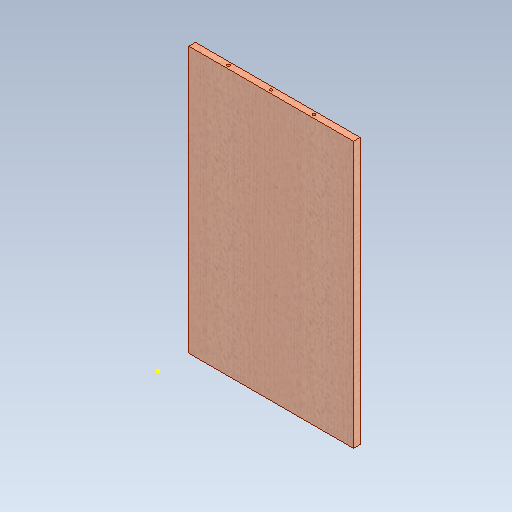
# Autodesk Inventor part: LateralInteriorCajoneras
Saved by Autodesk Inventor 2020.3 (Build 243373000, 373)
## iProperties
Created: 2020-10-30
Part Number: LateralInteriorCajoneras
Material: Madera (roble)
Document SubType Name: Modeling
Designer: codig
Density: 0.76 g/cm^3
Appearance: Roble blanco - Natural brillo medio
Author: codig
Autodesk Inventor part; units mm, degrees
ref_plane "YZ Plane" through (0, 0, 0) normal (1, 0, 0) x (0, 1, 0)
ref_plane "XZ Plane" through (0, 0, 0) normal (0, 1, 0) x (-1, 0, 0)
ref_plane "XY Plane" through (0, 0, 0) normal (0, 0, 1) x (1, 0, 0)
sketch "Boceto1" plane through (0, 0, 0) normal (0, 0, 1) x (1, 0, 0)
  line L0 (100, 100) -> (546, 100)
  line L1 (546, 100) -> (546, 820)
  line L2 (546, 820) -> (100, 820)
  line L3 (100, 820) -> (100, 100)
  point P0 (0, 0)
  constraints: 8 end point, 2 parallel, 1 horizontal, 1 perpendicular
extrude "Extrusión1" add sketch "Boceto1" along normal blind 18
sketch "Boceto2" plane through (100, 100, 0) normal (-1, 0, 0) x (0, 0, 1)
  line L0 (0, 0) -> (18, 0) projected
  line L1 (0, 0) -> (0, 720) projected
  circle A0 centre (9, 180) radius 4
  circle A1 centre (9, 360) radius 4
  circle A2 centre (9, 540) radius 4
  point P0 (0, -100)
  constraints: 3 centre point
hole "Agujero1" at (100, 640, 9) at (100, 460, 9) at (100, 280, 9) direction (1, 0, 0) diameter 8 depth 35
sketch "Boceto3" plane through (100, 820, 0) normal (0, 1, 0) x (1, 0, 0)
  line L0 (446, 0) -> (446, -18) projected
  circle A0 centre (214, -9) radius 4
  circle A1 centre (98, -9) radius 4
  circle A2 centre (330, -9) radius 4
  point P0 (-100, 0)
  constraints: 3 centre point
hole "Agujero2" at (430, 820, 9) at (314, 820, 9) at (198, 820, 9) direction (0, -1, 0) diameter 8 depth 35
sketch "Boceto4" plane through (0, 0, 0) normal (0, 0, -1) x (-1, 0, 0)
  circle A0 centre (-430, 129) radius 4
  circle A1 centre (-314, 129) radius 4
  circle A2 centre (-198, 129) radius 4
  point P0 (0, 0)
  constraints: 3 centre point
hole "Agujero3" at (430, 129, 0) at (314, 129, 0) at (198, 129, 0) direction (0, 0, 1) diameter 8 depth 10
sketch "Boceto5" plane through (0, 0, 0) normal (0, 0, -1) x (-1, 0, 0)
  point P0 (0, 0)
sketch "Boceto6" plane through (0, 0, 0) normal (0, 0, -1) x (-1, 0, 0)
  line L0 (-135, 456) -> (-135, 464) projected
  line L1 (-546, 100) -> (-546, 820) projected
  circle A0 centre (-430, 129) radius 4 projected
  circle A1 centre (-314, 129) radius 4 projected
  circle A2 centre (-198, 129) radius 4 projected
  circle A3 centre (-430, 460) radius 4
  circle A4 centre (-314, 460) radius 4
  circle A5 centre (-198, 460) radius 4
  point P0 (0, 0)
  constraints: 3 centre point
hole "Agujero4" at (430, 460, 0) at (314, 460, 0) at (198, 460, 0) direction (0, 0, 1) diameter 8 depth 10
sketch "Boceto7" plane through (100, 100, 0) normal (0, -1, 0) x (1, 0, 0)
  circle A0 centre (330, 9) radius 4
  circle A1 centre (214, 9) radius 4
  circle A2 centre (98, 9) radius 4
  point P0 (-100, 0)
  constraints: 3 centre point
hole "Agujero5" at (430, 100, 9) at (314, 100, 9) at (198, 100, 9) direction (0, 1, 0) diameter 8 depth 23
